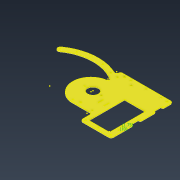
# Autodesk Inventor part: wstepna_geometria_wersja_2
Saved by Autodesk Inventor 2022.3 (Build 263350030, 350C)
## iProperties
Created: 2022-02-09
Part Number: wstepna_geometria_wersja_2
Material: Aluminum 6061
Document SubType Name: Modeling
Designer: Tomasz Krakowski
Density: 2.7 g/cm^3
Appearance: Kanarkowa
Mass: 61.75 g
Surface Area: 250.249 cm^2
Volume: 22.8704 cm^3
Author: Tomasz Krakowski
Autodesk Inventor part; units mm, degrees
ref_plane "YZ Plane" through (0, 0, 0) normal (1, 0, 0) x (0, 1, 0)
ref_plane "XZ Plane" through (0, 0, 0) normal (0, 1, 0) x (-1, 0, 0)
ref_plane "XY Plane" through (0, 0, 0) normal (0, 0, 1) x (1, 0, 0)
sketch "Sketch1" plane through (0, 0, 0) normal (0, 1, 0) x (-1, 0, 0)
  arc A0 (-0.3814, 2.9757) -> (-3, 0) centre (0, 0) ccw
  arc A1 (-0.3814, 2.9757) -> (0, 75) centre (-5, 39.0133) ccw
  line L0 (-105, 0) -> (0, 0) construction
  line L1 (-3, 0) -> (-105, 0) construction
  arc A2 (-3, 0) -> (-0.3814, -2.9757) centre (0, 0) ccw
  arc A3 (-1.6619, -2.4976) -> (97.0992, -0.9275) centre (46.5785, 70) ccw
  arc A4 (102.9008, -9.0725) -> (97.0992, -0.9275) centre (100, -5) ccw
  line L2 (0, 0) -> (100, 0) construction
  arc A5 (5.6849, -18.0476) -> (102.9008, -9.0725) centre (46.5785, 70) ccw
  line L3 (0, 75) -> (0, 0) construction
  line L4 (0, 0) -> (0, -15.1769) construction
  line L5 (0, 0) -> (-105, 0) construction
  line L6 (0, 75) -> (-105, 75)
  line L7 (-105, 75) -> (-105, -25)
  line L8 (0, -21.6754) -> (0, -21)
  line L9 (-4, -25) -> (-105, -25)
  arc A6 (5.6849, -18.0476) -> (0, -21.6754) centre (4, -21.6754) ccw
  arc A7 (-4, -25) -> (0, -21) centre (-4, -21) ccw
  circle A8 centre (-5, 35) radius 11
  point P0 (-5, -39.0133)
  point P1 (0, -25)
  dimension "d0" = 6
  dimension "d13" = 5
  dimension "d47" = 10
  dimension "d48" = 100
  dimension "d49" = 100
  dimension "d68" = 70
  dimension "d71" = 0
  dimension "d73" = 25
  dimension "d75" = 105
  dimension "d76" = 4
  dimension "d77" = 4
  dimension "d101" = 22
  dimension "d102" = 5
  dimension "d103" = 35
  dimension "d108" = 75
  constraints: 20 end point, 18 point on circle, 9 centre point, 9 tangent, 6 point on line, 5 horizontal, 3 coincident, 2 symmetric about line, 2 vertical, 1 collinear, 1 perpendicular, 1 other
  measures "d0" diameter of A0
  measures "d13" horizontal distance of point (0, 0) A1.centre
  measures "d47" diameter of A4
  measures "d48" distance of L2.end point (0, 0)
  measures "d49" horizontal distance of point (0, 0) A4.centre
  measures "d68" vertical distance of point (0, 0) A3.centre
  measures "d71" distance between parallel lines of L5 L1
  measures "d73" distance from line of L9 point (0, 0)
  measures "d75" horizontal distance of point (0, 0) L6.end
  measures "d76" radius of A6
  measures "d77" radius of A7
  measures "d101" diameter of A8
  measures "d102" horizontal distance of point (0, 0) A8.centre
  measures "d103" vertical distance of A8.centre point (0, 0)
  measures "d108" distance from line of L6 point (0, 0)
extrude "Extrusion1" add sketch "Sketch1" along normal blind 2
sketch "Szkic5" plane through (0, 2, 0) normal (0, 1, 0) x (1, 0, 0)
  circle A0 centre (12.5, -67.5) radius 2.1
  circle A1 centre (97.5, -67.5) radius 2.1
  line L0 (97.5, -67.5) -> (97.5, 52.5) construction
  line L1 (12.5, -67.5) -> (97.5, -67.5) construction
  line L2 (0, -75) -> (105, -75) construction
  line L3 (105, -75) -> (105, 25) construction
  line L4 (105, 25) -> (4, 25) construction
  line L5 (0, 21) -> (0, 21.6754) construction
  circle A2 centre (97.5, 20) radius 2.1
  circle A3 centre (12.5, 20) radius 2.1
  line L6 (12.5, 20) -> (97.5, 20) construction
  point P0 (0, 0)
  dimension "d84" = 7.5
  dimension "d85" = 7.5
  dimension "d89" = 85
  dimension "d106" = 87.5
  dimension "d107" = 85
  dimension "d109" = 4.2
  constraints: 6 end point, 4 centre point, 3 equal radius, 1 horizontal, 1 perpendicular, 1 point on line, 1 vertical
  measures "d84" distance between parallel lines of L2 L1
  measures "d85" distance between parallel lines of L3 L0
  measures "d89" distance of L1.start L0.start
  measures "d106" distance between parallel lines of L1 L6
  measures "d107" distance of L6.start L6.end
  measures "d109" diameter of A3
extrude "Wyciągnięcie proste4" cut sketch "Szkic5" against normal up to surface (2 mm away)
sketch "Szkic6" plane through (0, 2, 0) normal (0, 1, 0) x (1, 0, 0)
  line L0 (105, -55) -> (100.9, -55)
  line L1 (100.9, -55) -> (100.9, -40)
  line L2 (100.9, -40) -> (105, -40)
  line L3 (105, -40) -> (105, -55)
  line L4 (105, -10) -> (100.9, -10)
  line L5 (100.9, -10) -> (100.9, 5)
  line L6 (100.9, 5) -> (105, 5)
  line L7 (105, 5) -> (105, -10)
  line L8 (100.9, -40) -> (100.9, -10) construction
  line L9 (105, -75) -> (105, 25) construction
  line L10 (100.9, -25) -> (105, -25) construction
  point P0 (0, 0)
  dimension "d92" = 15
  dimension "d94" = 30
  dimension "d134" = 4.1
  constraints: 20 end point, 5 parallel, 3 collinear, 3 perpendicular, 2 horizontal, 2 midpoint, 1 point on line
  measures "d92" distance of L4.end L5.end
  measures "d94" distance between parallel lines of L4 L2
  measures "d134" distance between parallel lines of L9 L1
extrude "Wyciągnięcie proste5" cut sketch "Szkic6" against normal up to surface (2 mm away)
sketch "Sketch9" plane through (0, 2, 0) normal (0, 1, 0) x (1, 0, 0)
  line L0 (-11.5, -35) -> (21.5, -35) construction
  circle A0 centre (-11.5, -35) radius 1.6
  circle A1 centre (21.5, -35) radius 1.6
  circle A2 centre (5, -35) radius 11 construction
  point P0 (0, 0)
  dimension "d110" = 33
  dimension "d111" = 3.2
  constraints: 3 coincident, 2 centre point, 2 end point, 1 equal radius, 1 horizontal, 1 midpoint
  measures "d110" distance of L0.start L0.end
  measures "d111" diameter of A0
extrude "Extrusion6" cut sketch "Sketch9" against normal through all
fillet "Fillet1" radius 5 1 edges at (105, 1, -25)
sketch "Sketch10" plane through (0, 2, 0) normal (0, 1, 0) x (1, 0, 0)
  circle A0 centre (6, 12.5) radius 1.75
  circle A1 centre (34, 12.5) radius 1.75
  line L0 (6, 12.5) -> (34, 12.5) construction
  line L1 (100, 25) -> (4, 25) construction
  point P0 (0, 0)
  dimension "d115" = 3.5
  dimension "d116" = 28
  dimension "d117" = 12.5
  dimension "d118" = 6
  constraints: 2 centre point, 2 end point, 1 equal radius, 1 horizontal
  measures "d115" diameter of A0
  measures "d116" distance of L0.end L0.start
  measures "d117" distance between parallel lines of L1 L0
  measures "d118" horizontal distance of L0.start point (0, 0)
extrude "Extrusion7" cut sketch "Sketch10" against normal through all
sketch "Sketch11" plane through (0, 2, 0) normal (0, 1, 0) x (1, 0, 0)
  line L0 (93.5, -75) -> (51.5, -75)
  line L1 (51.5, -75) -> (51.5, -18)
  line L2 (51.5, -18) -> (93.5, -18)
  line L3 (93.5, -18) -> (93.5, -75)
  line L4 (0, -75) -> (105, -75) construction
  point P0 (0, 0)
  point P1 (100, -75)
  dimension "d121" = 42
  dimension "d122" = 57
  dimension "d123" = 51.5
  constraints: 8 end point, 2 parallel, 1 collinear, 1 horizontal, 1 perpendicular
  measures "d121" distance of L1.end L2.end
  measures "d122" distance between parallel lines of L0 L2
  measures "d123" distance from line of point (0, 0) L1
extrude "Extrusion8" cut sketch "Sketch11" against normal through all
sketch "Sketch12" plane through (0, 2, 0) normal (0, 1, 0) x (1, 0, 0)
  line L0 (93.5, -75) -> (105, -75) projected
  line L1 (93.5, -75) -> (93.5, -90.5)
  line L2 (93.5, -90.5) -> (51.5, -90.5)
  line L3 (0, -75) -> (51.5, -75) projected
  line L4 (51.5, -90.5) -> (51.5, -75)
  line L5 (93.5, -75) -> (105, -75)
  line L6 (105, -75) -> (105, -98.5)
  line L7 (105, -98.5) -> (43.5, -98.5)
  line L8 (43.5, -98.5) -> (43.5, -75)
  point P0 (0, 0)
  dimension "d126" = 15.5
  dimension "d127" = 8
  dimension "d128" = 8
  constraints: 14 end point, 4 perpendicular, 2 vertical, 1 horizontal, 1 point on line
  measures "d126" distance from line of L0.start L2
  measures "d127" distance between parallel lines of L7 L2
  measures "d128" distance between parallel lines of L8 L4
extrude "Extrusion9" add sketch "Sketch12" against normal up to surface (2 mm away)
fillet "Fillet2" radius 5 3 edges at (43.5, 1, 75) (43.5, 1, 98.5) (105, 1, 98.5)
fillet "Fillet3" radius 1 4 edges at (51.5, 1, 18) (93.5, 1, 18) (93.5, 1, 90.5) (51.5, 1, 90.5)
fillet "Fillet4" radius 2 4 edges at (105, 1, 55) (105, 1, 40) (105, 1, 10) (105, 1, -5)
sketch "Sketch13" plane through (0, 2, 0) normal (0, 1, 0) x (1, 0, 0)
  line L0 (99.25, -77.5) -> (99.25, -93.5) construction
  line L1 (93.5, -19) -> (93.5, -89.5) construction
  line L2 (93.5, -89.5) -> (105, -89.5) construction
  line L3 (105, -93.5) -> (105, -57) construction
  point P0 (0, 0)
  point P1 (99.25, -89.5)
  dimension "d137" = 12
  dimension "d138" = 4
  constraints: 4 end point, 2 coincident, 2 point on line, 1 midpoint, 1 perpendicular, 1 vertical
  measures "d137" distance from line of L2 L0.start
  measures "d138" distance of L0.end point (99.25, -89.5)
hole "Hole1" at (99.25, 2, 77.5) at (99.25, 2, 93.5) direction (0, -1, 0) diameter 3.2 end through all
sketch "Sketch14" plane through (0, 2, 0) normal (0, 1, 0) x (1, 0, 0)
  arc A0 (1.6619, 2.4976) -> (-97.0992, 0.9275) centre (-46.5785, -70) ccw construction
  arc A1 (-102.9008, 9.0725) -> (-97.0992, 0.9275) centre (-100, 5) ccw projected
  arc A2 (13.245, 0) -> (-100, 5) centre (-46.5785, -70) ccw construction
  line L0 (0, 0) -> (13.245, 0) construction
  line L1 (-46.5785, -70) -> (-100, 5) construction
  line L2 (24.9599, 21) -> (84.9599, 21) construction
  circle A3 centre (12.5, 20) radius 2.1 projected
  circle A4 centre (97.5, 20) radius 2.1 projected
  line L3 (100, 25) -> (4, 25) projected
  line L4 (0, -70) -> (38.5, -70) construction
  arc A5 (43.5, -80) -> (38.5, -75) centre (38.5, -80) ccw projected
  line L5 (38.5, -70) -> (38.5, -75) construction
  line L6 (0, -75) -> (0, -70) construction
  line L7 (0, -75) -> (38.5, -75) projected
  arc A6 (100, -98.5) -> (105, -93.5) centre (100, -93.5) ccw projected
  line L8 (48.5, -93.5) -> (100, -93.5) construction
  arc A7 (43.5, -93.5) -> (48.5, -98.5) centre (48.5, -93.5) ccw construction
  arc A8 (100, -98.5) -> (105, -93.5) centre (100, -93.5) ccw construction
  point P0 (54.9599, 21)
  point P1 (74.25, -93.5)
  point P2 (-78.7683, 16.2709)
  point P3 (-78.7683, 16.2709)
  point P4 (-78.7683, 16.2709)
  point P5 (-55.3429, 21.6626)
  point P6 (-55.3429, 21.6626)
  point P7 (-55.3429, 21.6626)
  point P8 (-31.3202, 20.8077)
  point P9 (-31.3202, 20.8077)
  point P10 (-31.3202, 20.8077)
  point P11 (-8.3374, 13.7643)
  point P12 (-8.3374, 13.7643)
  point P13 (-8.3374, 13.7643)
  dimension "d150" = 60
  dimension "d151" = 12.5
  dimension "d152" = 4
  dimension "d153" = 5
  dimension "d156" = 60
  constraints: 14 end point, 12 coincident, 3 horizontal, 2 midpoint, 2 perpendicular, 2 point on circle, 1 centre point, 13 other
  measures "d150" distance of L2.start L2.end
  measures "d151" distance of point (24.96, 21) A3.centre
  measures "d152" distance between parallel lines of L3 L2
  measures "d153" distance between parallel lines of L7 L4
hole "Hole2" at (-100, 2, -5) at (24.9599, 2, -21) at (54.9599, 2, -21) at (84.9599, 2, -21) at (0, 2, 70) at (38.5, 2, 70) at (48.5, 2, 93.5) at (74.25, 2, 93.5) at (-78.7683, 2, -16.2709) at (-55.3429, 2, -21.6626) at (-31.3202, 2, -20.8077) at (-8.3374, 2, -13.7643) direction (0, -1, 0) diameter 3.2 end through all
sketch "Sketch15" plane through (0, 2, 0) normal (0, 1, 0) x (1, 0, 0)
  line L0 (30, -40) -> (31.5, -40)
  line L1 (31.5, -40) -> (31.5, -51)
  line L2 (31.5, -51) -> (30, -51)
  line L3 (30, -51) -> (30, -40)
  line L4 (41.5, -40) -> (43, -40)
  line L5 (43, -40) -> (43, -51)
  line L6 (43, -51) -> (41.5, -51)
  line L7 (41.5, -51) -> (41.5, -40)
  point P0 (0, 0)
  dimension "d165" = 1.5
  dimension "d166" = 11
  dimension "d167" = 10
  dimension "d168" = 40
  dimension "d169" = 30
  constraints: 16 end point, 4 parallel, 2 horizontal, 2 perpendicular, 2 point on line, 1 collinear
  measures "d165" distance of L0.start L0.end
  measures "d166" vertical distance of L5.end L4.start
  measures "d167" distance between parallel lines of L7 L1
  measures "d168" vertical distance of point (0, 0) L0.start
  measures "d169" distance from line of L3 point (0, 0)
extrude "Extrusion10" cut sketch "Sketch15" against normal through all
sketch "Sketch16" plane through (0, 2, 0) normal (0, 1, 0) x (1, 0, 0)
  line L0 (43, -40) -> (43, -51) projected
  line L1 (43, -51) -> (41.5, -51) projected
  line L2 (41.5, -51) -> (41.5, -40) projected
  line L3 (41.5, -40) -> (43, -40) projected
  line L4 (31.5, -40) -> (31.5, -51) projected
  line L5 (31.5, -51) -> (30, -51) projected
  line L6 (30, -51) -> (30, -40) projected
  line L7 (30, -40) -> (31.5, -40) projected
  circle A0 centre (-31.3202, 20.8077) radius 1.6 projected
  circle A1 centre (-78.7683, 16.2709) radius 1.6 projected
  circle A2 centre (48.5, -93.5) radius 1.6 projected
  circle A3 centre (0, -70) radius 1.6 projected
  circle A4 centre (54.9599, 21) radius 1.6 projected
  circle A5 centre (-100, 5) radius 1.6 projected
  circle A6 centre (24.9599, 21) radius 1.6 projected
  circle A7 centre (84.9599, 21) radius 1.6 projected
  circle A8 centre (38.5, -70) radius 1.6 projected
  circle A9 centre (74.25, -93.5) radius 1.6 projected
  circle A10 centre (-55.3429, 21.6626) radius 1.6 projected
  circle A11 centre (-8.3374, 13.7643) radius 1.6 projected
  circle A12 centre (99.25, -77.5) radius 1.6 projected
  circle A13 centre (99.25, -93.5) radius 1.6 projected
  line L8 (51.5, -89.5) -> (51.5, -19) projected
  arc A14 (52.5, -18) -> (51.5, -19) centre (52.5, -19) ccw projected
  line L9 (52.5, -18) -> (92.5, -18) projected
  arc A15 (93.5, -19) -> (92.5, -18) centre (92.5, -19) ccw projected
  line L10 (93.5, -19) -> (93.5, -89.5) projected
  arc A16 (92.5, -90.5) -> (93.5, -89.5) centre (92.5, -89.5) ccw projected
  line L11 (92.5, -90.5) -> (52.5, -90.5) projected
  arc A17 (51.5, -89.5) -> (52.5, -90.5) centre (52.5, -89.5) ccw projected
  circle A18 centre (34, 12.5) radius 1.75 projected
  circle A19 centre (6, 12.5) radius 1.75 projected
  circle A20 centre (-11.5, -35) radius 1.6 projected
  circle A21 centre (21.5, -35) radius 1.6 projected
  circle A22 centre (97.5, 20) radius 2.1 projected
  circle A23 centre (12.5, 20) radius 2.1 projected
  circle A24 centre (97.5, -67.5) radius 2.1 projected
  circle A25 centre (12.5, -67.5) radius 2.1 projected
  circle A26 centre (5, -35) radius 11 projected
  arc A27 (103, 5) -> (105, 7) centre (103, 7) ccw projected
  line L12 (105, 7) -> (105, 20) projected
  arc A28 (105, 20) -> (100, 25) centre (100, 20) ccw projected
  line L13 (100, 25) -> (4, 25) projected
  arc A29 (4, 25) -> (0, 21) centre (4, 21) ccw projected
  line L14 (0, 21) -> (0, 21.6754) projected
  arc A30 (-5.6849, 18.0476) -> (0, 21.6754) centre (-4, 21.6754) ccw projected
  arc A31 (-5.6849, 18.0476) -> (-102.9008, 9.0725) centre (-46.5785, -70) ccw projected
  arc A32 (-102.9008, 9.0725) -> (-97.0992, 0.9275) centre (-100, 5) ccw projected
  arc A33 (1.6619, 2.4976) -> (-97.0992, 0.9275) centre (-46.5785, -70) ccw projected
  arc A34 (0.3814, -2.9757) -> (1.6619, 2.4976) centre (0, 0) ccw projected
  arc A35 (0.3814, -2.9757) -> (0, -75) centre (5, -39.0133) ccw projected
  line L15 (0, -75) -> (38.5, -75) projected
  arc A36 (43.5, -80) -> (38.5, -75) centre (38.5, -80) ccw projected
  line L16 (43.5, -80) -> (43.5, -93.5) projected
  arc A37 (43.5, -93.5) -> (48.5, -98.5) centre (48.5, -93.5) ccw projected
  line L17 (48.5, -98.5) -> (100, -98.5) projected
  arc A38 (100, -98.5) -> (105, -93.5) centre (100, -93.5) ccw projected
  line L18 (105, -93.5) -> (105, -57) projected
  arc A39 (105, -57) -> (103, -55) centre (103, -57) ccw projected
  line L19 (103, -55) -> (100.9, -55) projected
  line L20 (100.9, -55) -> (100.9, -40) projected
  line L21 (100.9, -40) -> (103, -40) projected
  arc A40 (103, -40) -> (105, -38) centre (103, -38) ccw projected
  line L22 (105, -38) -> (105, -12) projected
  arc A41 (105, -12) -> (103, -10) centre (103, -12) ccw projected
  line L23 (103, -10) -> (100.9, -10) projected
  line L24 (100.9, -10) -> (100.9, 5) projected
  line L25 (100.9, 5) -> (103, 5) projected
  point P0 (0, 0)
  dimension "d172" = 10
  dimension "d173" = 1.75
  measures "d172" vertical distance of A24.centre A12.centre
  measures "d173" horizontal distance of A24.centre A12.centre
body "Solid1"
